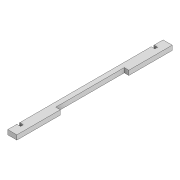
# Autodesk Inventor part: Gel top
Saved by Autodesk Inventor 2020 (Build 240168000, 168)
## iProperties
Created: 2022-04-26
Part Number: Gel top
Material: Generic
Document SubType Name: Modeling
Designer: ferrerx
Density: 1 g/cm^3
Appearance: Default
Author: ferrerx
Autodesk Inventor part; units mm, degrees
ref_plane "YZ Plane" through (0, 0, 0) normal (1, 0, 0) x (0, 1, 0)
ref_plane "XZ Plane" through (0, 0, 0) normal (0, 1, 0) x (-1, 0, 0)
ref_plane "XY Plane" through (0, 0, 0) normal (0, 0, 1) x (1, 0, 0)
sketch "Sketch1" plane through (0, 0, 0) normal (0, 1, 0) x (-1, 0, 0)
  line L0 (5, 85) -> (-5, 85)
  line L1 (-5, 85) -> (-5, -85)
  line L2 (-5, -85) -> (5, -85)
  line L3 (5, -85) -> (5, 85)
  line L4 (5, 85) -> (-5, -85) construction
  line L5 (-5, 85) -> (5, -85) construction
  point P0 (0, 0)
  dimension "d0" = 170
  dimension "d1" = 10
  constraints: 12 end point, 2 midpoint, 2 parallel, 1 horizontal, 1 perpendicular
  measures "d0" distance of L2.end L0.start
  measures "d1" distance of L1.end L2.end
extrude "Extrusion1" add sketch "Sketch1" along normal blind 5
sketch "Sketch2" plane through (0, 5, 0) normal (0, 1, 0) x (1, 0, 0)
  line L0 (-5, 85) -> (-5, -85) projected
  line L1 (-5, -75) -> (-1, -75)
  line L2 (-1, -75) -> (-1, -72)
  line L3 (-1, -72) -> (-5, -72)
  line L4 (-5, -72) -> (-5, -75)
  line L5 (-5, -85) -> (5, -85) projected
  line L6 (5, 0) -> (-5, 0) construction
  line L7 (-5, 75) -> (-1, 75)
  line L8 (-1, 75) -> (-1, 72)
  line L9 (-1, 72) -> (-5, 72)
  line L10 (-5, 72) -> (-5, 75)
  point P0 (0, 0)
  point P1 (-5, 75)
  point P2 (-5, 72)
  dimension "d4" = 3
  dimension "d5" = 4
  dimension "d6" = 10
  constraints: 18 end point, 4 symmetric about line, 2 parallel, 1 horizontal, 1 midpoint, 1 perpendicular, 1 point on line
  measures "d4" distance between parallel lines of L1 L3
  measures "d5" distance of L1.start L1.end
  measures "d6" distance between parallel lines of L5 L1
extrude "Extrusion2" cut sketch "Sketch2" against normal blind 5
sketch "Sketch3" plane through (0, 5, 0) normal (0, 1, 0) x (1, 0, 0)
  line L0 (0, 37.5) -> (10, 37.5)
  line L1 (10, 37.5) -> (10, -37.5)
  line L2 (10, -37.5) -> (0, -37.5)
  line L3 (0, -37.5) -> (0, 37.5)
  line L4 (5, -85) -> (5, 85) projected
  line L5 (0, 37.5) -> (10, -37.5) construction
  line L6 (10, 37.5) -> (0, -37.5) construction
  point P0 (0, 0)
  point P1 (5, 0)
  point P2 (5, -37.5)
  point P3 (5, 37.5)
  dimension "d9" = 75
  dimension "d10" = 5
  constraints: 12 end point, 3 midpoint, 2 parallel, 1 horizontal, 1 perpendicular
  measures "d9" distance of L0.end L1.end
  measures "d10" distance between parallel lines of L4 L3
extrude "Extrusion3" cut sketch "Sketch3" against normal blind 10 contours L0 L4 L2 L3
body "Solid1"
